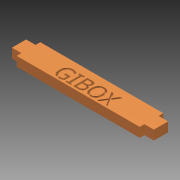
# Autodesk Inventor part: frontal mes nom
Saved by Autodesk Inventor 2012 SP1 (Build 160190100, 190)
## iProperties
Created: 2014-12-30
Part Number: frontal mes nom
Material: Default
Document SubType Name: Modeling
Designer: PRINCIPAL
Density: 1 g/cm^3
Author: PRINCIPAL
Autodesk Inventor part; units mm, degrees
ref_plane "YZ Plane" through (0, 0, 0) normal (1, 0, 0) x (0, 1, 0)
ref_plane "XZ Plane" through (0, 0, 0) normal (0, 1, 0) x (-1, 0, 0)
ref_plane "XY Plane" through (0, 0, 0) normal (0, 0, 1) x (1, 0, 0)
sketch "Boceto1" plane through (0, 0, 0) normal (0, 0, 1) x (1, 0, 0)
  line L0 (0, 0) -> (130, 0)
  line L1 (130, 0) -> (130, -25)
  line L2 (130, -25) -> (0, -25)
  line L3 (0, -25) -> (0, 0)
  dimension "d0" = 130
  dimension "d1" = 25
  constraints: 8 end point, 2 parallel, 1 horizontal, 1 perpendicular
  measures "d0" distance of L1.end L2.end
  measures "d1" distance between parallel lines of L2 L0
extrude "Extrusión1" add sketch "Boceto1" along normal blind 10
sketch "Boceto2" plane through (0, 0, 10) normal (0, 0, 1) x (1, 0, 0)
  line L0 (130, 0) -> (130, -25) projected
  line L1 (0, -25) -> (0, 0) projected
  line L2 (130, -25) -> (0, -25) projected
  line L3 (0, -5) -> (-10, -5)
  line L4 (-10, -5) -> (-10, -20)
  line L5 (-10, -20) -> (0, -20)
  line L6 (0, -20) -> (0, -5)
  line L7 (130, -5) -> (140, -5)
  line L8 (140, -5) -> (140, -20)
  line L9 (140, -20) -> (130, -20)
  line L10 (130, -20) -> (130, -5)
  dimension "d4" = 10
  dimension "d5" = 10
  dimension "d6" = 15
  dimension "d7" = 15
  dimension "d8" = 5
  dimension "d9" = 5
  constraints: 16 end point, 4 parallel, 2 horizontal, 2 perpendicular, 2 point on line
  measures "d4" distance of L5.end L4.end
  measures "d5" distance of L8.end L9.end
  measures "d6" distance between parallel lines of L5 L3
  measures "d7" distance between parallel lines of L9 L7
  measures "d8" distance between parallel lines of L5 L2
  measures "d9" distance from line of L0.end L9
extrude "Extrusión2" add sketch "Boceto2" against normal blind 10
sketch "Boceto3" plane through (0, 0, 10) normal (0, 0, 1) x (1, 0, 0)
  line L0 (15.2757, -7.5573) -> (105.0458, -7.5573) construction
  line L1 (105.0458, -7.5573) -> (105.0458, -28.4645) construction
  line L2 (105.0458, -28.4645) -> (15.2757, -28.4645) construction
  line L3 (15.2757, -28.4645) -> (15.2757, -7.5573) construction
  spline S0 degree 2 poles (42.407, -23.1651) (40.8146, -23.1651) (38.1769, -22.1926) (37.2287, -21.208) knots 0 0 0 1 2 2 2
  spline S1 degree 2 poles (37.2287, -21.208) (36.2806, -20.2113) (35.2717, -17.2696) (35.2717, -15.3612) knots 0 0 0 1 2 2 2
  spline S2 degree 2 poles (35.2717, -15.3612) (35.2717, -13.55) (36.2928, -10.6813) (37.2409, -9.6602) knots 0 0 0 1 2 2 2
  spline S3 degree 2 poles (37.2409, -9.6602) (38.1526, -8.6756) (40.8268, -7.6059) (42.4192, -7.6059) knots 0 0 0 1 2 2 2
  spline S4 degree 2 poles (42.4192, -7.6059) (43.185, -7.6059) (44.5707, -7.8247) (45.2028, -8.0192) knots 0 0 0 1 2 2 2
  spline S5 degree 2 poles (45.2028, -8.0192) (45.7133, -8.1651) (46.9532, -8.6999) (47.33, -8.8944) knots 0 0 0 1 2 2 2
  line L4 (47.33, -8.8944) -> (47.33, -11.3012)
  line L5 (47.33, -11.3012) -> (47.1599, -11.3012)
  spline S6 degree 2 poles (47.1599, -11.3012) (46.783, -10.973) (45.9929, -10.3774) (45.2636, -10.0371) knots 0 0 0 1 2 2 2
  spline S7 degree 2 poles (45.2636, -10.0371) (44.6558, -9.7332) (43.0877, -9.332) (42.1882, -9.332) knots 0 0 0 1 2 2 2
  spline S8 degree 2 poles (42.1882, -9.332) (40.0245, -9.332) (37.3503, -12.5897) (37.3503, -15.3004) knots 0 0 0 1 2 2 2
  spline S9 degree 2 poles (37.3503, -15.3004) (37.3503, -16.8077) (38.0553, -19.0687) (38.7239, -19.8466) knots 0 0 0 1 2 2 2
  spline S10 degree 2 poles (38.7239, -19.8466) (39.3681, -20.6246) (41.1915, -21.439) (42.3341, -21.439) knots 0 0 0 1 2 2 2
  spline S11 degree 2 poles (42.3341, -21.439) (43.1728, -21.439) (44.8503, -21.1959) (45.4216, -20.9528) knots 0 0 0 1 2 2 2
  line L6 (45.4216, -20.9528) -> (45.4216, -17.0751)
  line L7 (45.4216, -17.0751) -> (41.9451, -17.0751)
  line L8 (41.9451, -17.0751) -> (41.9451, -15.3247)
  line L9 (41.9451, -15.3247) -> (47.3908, -15.3247)
  line L10 (47.3908, -15.3247) -> (47.3908, -21.8766)
  spline S12 degree 2 poles (47.3908, -21.8766) (47.014, -22.0468) (45.7255, -22.5695) (45.1785, -22.7275) knots 0 0 0 1 2 2 2
  spline S13 degree 2 poles (45.1785, -22.7275) (44.437, -22.9463) (43.2458, -23.1651) (42.407, -23.1651) knots 0 0 0 1 2 2 2
  line L11 (55.1218, -22.8734) -> (49.3114, -22.8734)
  line L12 (49.3114, -22.8734) -> (49.3114, -21.3418)
  line L13 (49.3114, -21.3418) -> (51.2198, -21.3418)
  line L14 (51.2198, -21.3418) -> (51.2198, -9.405)
  line L15 (51.2198, -9.405) -> (49.3114, -9.405)
  line L16 (49.3114, -9.405) -> (49.3114, -7.8734)
  line L17 (49.3114, -7.8734) -> (55.1218, -7.8734)
  line L18 (55.1218, -7.8734) -> (55.1218, -9.405)
  line L19 (55.1218, -9.405) -> (53.2133, -9.405)
  line L20 (53.2133, -9.405) -> (53.2133, -21.3418)
  line L21 (53.2133, -21.3418) -> (55.1218, -21.3418)
  line L22 (55.1218, -21.3418) -> (55.1218, -22.8734)
  spline S14 degree 2 poles (67.7636, -18.2664) (67.7636, -19.3847) (66.9127, -21.0986) (66.2077, -21.6578) knots 0 0 0 1 2 2 2
  spline S15 degree 2 poles (66.2077, -21.6578) (65.3568, -22.3142) (63.424, -22.8734) (61.8924, -22.8734) knots 0 0 0 1 2 2 2
  line L23 (61.8924, -22.8734) -> (57.5894, -22.8734)
  line L24 (57.5894, -22.8734) -> (57.5894, -7.8734)
  line L25 (57.5894, -7.8734) -> (61.5642, -7.8734)
  spline S16 degree 2 poles (61.5642, -7.8734) (63.1688, -7.8734) (64.7733, -8.08) (65.5026, -8.4811) knots 0 0 0 1 2 2 2
  spline S17 degree 2 poles (65.5026, -8.4811) (66.3171, -8.9066) (67.0586, -10.3045) (67.0586, -11.2526) knots 0 0 0 1 2 2 2
  spline S18 degree 2 poles (67.0586, -11.2526) (67.0586, -12.3101) (65.9402, -13.9876) (64.9556, -14.4617) knots 0 0 0 1 2 2 2
  line L26 (64.9556, -14.4617) -> (64.9556, -14.5346)
  spline S19 degree 2 poles (64.9556, -14.5346) (66.2928, -14.8993) (67.7636, -16.832) (67.7636, -18.2664) knots 0 0 0 1 2 2 2
  spline S20 degree 2 poles (65.685, -18.3515) (65.685, -17.5006) (65.1988, -16.4066) (64.4694, -16.0176) knots 0 0 0 1 2 2 2
  spline S21 degree 2 poles (64.4694, -16.0176) (63.9954, -15.7745) (62.877, -15.6286) (61.8438, -15.6286) knots 0 0 0 1 2 2 2
  line L27 (61.8438, -15.6286) -> (59.5829, -15.6286)
  line L28 (59.5829, -15.6286) -> (59.5829, -21.1716)
  line L29 (59.5829, -21.1716) -> (61.1996, -21.1716)
  spline S22 degree 2 poles (61.1996, -21.1716) (62.5124, -21.1716) (64.0197, -20.9285) (64.6031, -20.5395) knots 0 0 0 1 2 2 2
  spline S23 degree 2 poles (64.6031, -20.5395) (65.1623, -20.1383) (65.685, -19.1416) (65.685, -18.3515) knots 0 0 0 1 2 2 2
  spline S24 degree 2 poles (64.98, -11.5322) (64.98, -10.9973) (64.6153, -10.1951) (64.2142, -9.9641) knots 0 0 0 1 2 2 2
  spline S25 degree 2 poles (64.2142, -9.9641) (63.7279, -9.6967) (62.5488, -9.5751) (61.4913, -9.5751) knots 0 0 0 1 2 2 2
  line L30 (61.4913, -9.5751) -> (59.5829, -9.5751)
  line L31 (59.5829, -9.5751) -> (59.5829, -13.9633)
  line L32 (59.5829, -13.9633) -> (61.8438, -13.9633)
  spline S26 degree 2 poles (61.8438, -13.9633) (62.7798, -13.9633) (63.6672, -13.7688) (64.1412, -13.4649) knots 0 0 0 1 2 2 2
  spline S27 degree 2 poles (64.1412, -13.4649) (64.6031, -13.1732) (64.98, -12.2372) (64.98, -11.5322) knots 0 0 0 1 2 2 2
  spline S28 degree 2 poles (80.3568, -9.5873) (81.2077, -10.5841) (82.1558, -13.5014) (82.1558, -15.3734) knots 0 0 0 1 2 2 2
  spline S29 degree 2 poles (82.1558, -15.3734) (82.1558, -17.1967) (81.232, -20.1505) (80.3568, -21.1473) knots 0 0 0 1 2 2 2
  spline S30 degree 2 poles (80.3568, -21.1473) (79.433, -22.1926) (76.9897, -23.1894) (75.5189, -23.1894) knots 0 0 0 1 2 2 2
  spline S31 degree 2 poles (75.5189, -23.1894) (73.9994, -23.1894) (71.5683, -22.1562) (70.6809, -21.1473) knots 0 0 0 1 2 2 2
  spline S32 degree 2 poles (70.6809, -21.1473) (69.8179, -20.1505) (68.8941, -17.221) (68.8941, -15.3734) knots 0 0 0 1 2 2 2
  spline S33 degree 2 poles (68.8941, -15.3734) (68.8941, -13.4892) (69.83, -10.6205) (70.6931, -9.5873) knots 0 0 0 1 2 2 2
  spline S34 degree 2 poles (70.6931, -9.5873) (71.5683, -8.5905) (74.0116, -7.5573) (75.5189, -7.5573) knots 0 0 0 1 2 2 2
  spline S35 degree 2 poles (75.5189, -7.5573) (77.0505, -7.5573) (79.5059, -8.627) (80.3568, -9.5873) knots 0 0 0 1 2 2 2
  spline S36 degree 2 poles (80.0772, -15.3734) (80.0772, -13.8904) (79.433, -11.593) (78.8495, -10.8393) knots 0 0 0 1 2 2 2
  spline S37 degree 2 poles (78.8495, -10.8393) (78.2539, -10.0614) (76.5764, -9.2834) (75.531, -9.2834) knots 0 0 0 1 2 2 2
  spline S38 degree 2 poles (75.531, -9.2834) (74.4492, -9.2834) (72.8203, -10.0371) (72.2004, -10.8393) knots 0 0 0 1 2 2 2
  spline S39 degree 2 poles (72.2004, -10.8393) (71.6048, -11.6051) (70.9727, -13.9147) (70.9727, -15.3734) knots 0 0 0 1 2 2 2
  spline S40 degree 2 poles (70.9727, -15.3734) (70.9727, -18.3272) (73.4524, -21.4633) (75.531, -21.4633) knots 0 0 0 1 2 2 2
  spline S41 degree 2 poles (75.531, -21.4633) (77.6096, -21.4633) (80.0772, -18.3272) (80.0772, -15.3734) knots 0 0 0 1 2 2 2
  line L33 (94.7125, -22.8734) -> (92.4273, -22.8734)
  line L34 (92.4273, -22.8734) -> (88.7806, -16.8928)
  line L35 (88.7806, -16.8928) -> (85.061, -22.8734)
  line L36 (85.061, -22.8734) -> (82.9095, -22.8734)
  line L37 (82.9095, -22.8734) -> (87.6866, -15.3612)
  line L38 (87.6866, -15.3612) -> (83.0553, -7.8734)
  line L39 (83.0553, -7.8734) -> (85.3406, -7.8734)
  line L40 (85.3406, -7.8734) -> (88.9143, -13.7445)
  line L41 (88.9143, -13.7445) -> (92.561, -7.8734)
  line L42 (92.561, -7.8734) -> (94.7125, -7.8734)
  line L43 (94.7125, -7.8734) -> (90.0205, -15.264)
  line L44 (90.0205, -15.264) -> (94.7125, -22.8734)
  constraints: 2 other
extrude "Extrusión3" cut sketch "Boceto3" against normal blind 4
